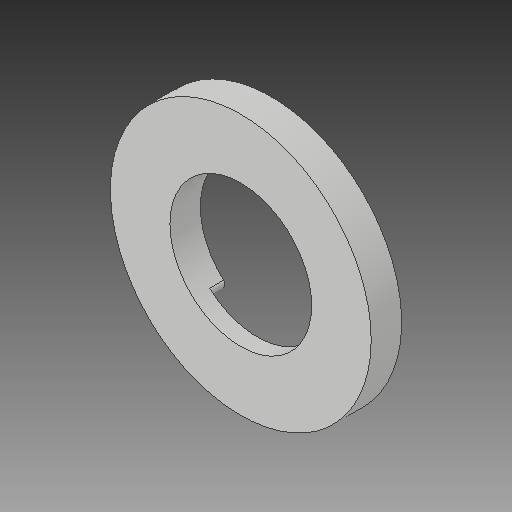
# Autodesk Inventor part: ヨー軸スペーサ
Saved by Autodesk Inventor 2017 (Build 210142000, 142)
## iProperties
Created: 2016-08-18
Part Number: ヨー軸スペーサ
Material: 一般
Document SubType Name: Modeling
Designer: NN
Density: 1 g/cm^3
Appearance: 既定
Mass: 1.53517 g
Surface Area: 14.7764 cm^2
Volume: 1.53517 cm^3
Author: NN
Autodesk Inventor part; units mm, degrees
ref_plane "YZ Plane" through (0, 0, 0) normal (1, 0, 0) x (0, 1, 0)
ref_plane "XZ Plane" through (0, 0, 0) normal (0, 1, 0) x (-1, 0, 0)
ref_plane "XY Plane" through (0, 0, 0) normal (0, 0, 1) x (1, 0, 0)
sketch "スケッチ1" plane through (0, 0, 0) normal (0, 0, 1) x (1, 0, 0)
  circle A0 centre (0, 0) radius 15
  dimension "d0" = 30
  constraints: 1 centre point, 1 coincident
  measures "d0" diameter of A0
extrude "押し出し1" add sketch "スケッチ1" along normal blind 3.5
sketch "スケッチ2" plane through (0, 0, 3.5) normal (0, 0, 1) x (1, 0, 0)
  circle A0 centre (0, 0) radius 4.05
  dimension "d3" = 8.1
  constraints: 1 centre point, 1 coincident
  measures "d3" diameter of A0
extrude "押し出し2" cut sketch "スケッチ2" against normal through all
sketch "スケッチ3" plane through (0, 0, 3.5) normal (0, 0, 1) x (1, 0, 0)
  circle A0 centre (0, 0) radius 8.15
  dimension "d6" = 16.3
  constraints: 1 centre point, 1 coincident
  measures "d6" diameter of A0
extrude "押し出し3" cut sketch "スケッチ3" against normal through all
sketch "スケッチ4" plane through (0, 0, 0) normal (0, 0, -1) x (-1, 0, 0)
  line L0 (-9.85, -6.9) -> (9.85, -6.9)
  line L1 (9.85, -6.9) -> (9.85, -21.9)
  line L2 (9.85, -21.9) -> (-9.85, -21.9)
  line L3 (-9.85, -21.9) -> (-9.85, -6.9)
  line L4 (0, -6.9) -> (0, 0)
  dimension "d9" = 19.7
  dimension "d10" = 6.9
  dimension "d11" = 15
  constraints: 10 end point, 2 parallel, 2 perpendicular, 1 horizontal, 1 midpoint
  measures "d9" distance of L1.end L2.end
  measures "d10" distance from line of L4.end L0
  measures "d11" distance between parallel lines of L0 L2
extrude "押し出し4" cut sketch "スケッチ4" against normal blind 1.6
fillet "フィレット2" radius 0.5 4 edges at (4.3373, -6.9, 0.8) (-4.3373, -6.9, 0.8) (9.85, -11.3127, 0.8) (-9.85, -11.3127, 0.8)
fillet "フィレット3" radius 1 2 edges at (-9.85, -6.9, 0.8) (9.85, -6.9, 0.8)
